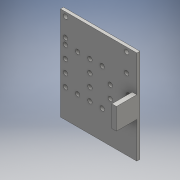
# Autodesk Inventor part: topChassis
Saved by Autodesk Inventor 2016 (Build 200138000, 138)
## iProperties
Created: 2016-05-01
Part Number: topChassis
Material: Generic
Document SubType Name: Modeling
Designer: mkepler
Density: 1 g/cm^3
Appearance: Default
Author: mkepler
Autodesk Inventor part; units mm, degrees
ref_plane "YZ Plane" through (0, 0, 0) normal (1, 0, 0) x (0, 1, 0)
ref_plane "XZ Plane" through (0, 0, 0) normal (0, 1, 0) x (-1, 0, 0)
ref_plane "XY Plane" through (0, 0, 0) normal (0, 0, 1) x (1, 0, 0)
sketch "Sketch1" plane through (0, 0, 0) normal (0, 1, 0) x (-1, 0, 0)
  line L0 (0, 0) -> (75, 0)
  line L1 (75, 0) -> (75, -92)
  line L2 (75, -92) -> (0, -92)
  line L3 (0, -92) -> (0, 0)
  line L4 (75, -46) -> (0, -46)
  circle A0 centre (70, -64) radius 2.175
  circle A1 centre (70, -28) radius 2.175
  circle A2 centre (58, -28) radius 2.175
  circle A3 centre (58, -64) radius 2.175
  circle A4 centre (46, -28) radius 2.175
  circle A5 centre (46, -64) radius 2.175
  circle A6 centre (34, -28) radius 2.175
  circle A7 centre (34, -64) radius 2.175
  dimension "d0" = 75
  dimension "d1" = 92
  dimension "d6" = 4.35
  dimension "d7" = 18
  dimension "d8" = 4.35
  dimension "d9" = 18
  dimension "d10" = 4.35
  dimension "d11" = 12
  dimension "d12" = 4.35
  dimension "d13" = 4.35
  dimension "d14" = 12
  dimension "d15" = 4.35
  dimension "d16" = 4.35
  dimension "d17" = 12
  dimension "d18" = 4.35
  dimension "d19" = 12
  dimension "d20" = 12
  dimension "d21" = 12
  constraints: 10 end point, 8 centre point, 2 midpoint, 2 parallel, 1 horizontal, 1 perpendicular
  measures "d0" distance of L1.end L2.end
  measures "d1" distance of L0.end L1.end
  measures "d6" diameter of A0
  measures "d7" distance from line of L4 A0.centre
  measures "d8" diameter of A1
  measures "d9" distance from line of L4 A1.centre
  measures "d10" diameter of A2
  measures "d11" distance of A2.centre A1.centre
  measures "d12" diameter of A3
  measures "d13" diameter of A4
  measures "d14" distance of A4.centre A2.centre
  measures "d15" diameter of A5
  measures "d16" diameter of A6
  measures "d17" distance of A4.centre A6.centre
  measures "d18" diameter of A7
  measures "d19" distance of A3.centre A0.centre
  measures "d20" distance of A5.centre A3.centre
  measures "d21" distance of A7.centre A5.centre
extrude "Extrusion1" add sketch "Sketch1" along normal blind 3
sketch "Sketch3" plane through (0, 0, 0) normal (0, -1, 0) x (1, 0, 0)
  line L0 (0, 0) -> (0, -92) projected
  line L1 (-4.5, -46) -> (-75, -46)
  line L2 (-75, -92) -> (-75, 0) projected
  line L3 (0, -46) -> (0, -56.5)
  line L4 (0, -56.5) -> (-4.5, -56.5)
  line L5 (-4.5, -56.5) -> (-4.5, -35.5)
  line L6 (-4.5, -35.5) -> (0, -35.5)
  line L7 (0, -56.5) -> (0, -35.5)
  dimension "d24" = 10.5
  dimension "d25" = 4.5
  dimension "d26" = 21
  constraints: 12 end point, 3 midpoint, 2 perpendicular, 2 point on line, 1 collinear, 1 vertical
  measures "d24" distance of L3.start L3.end
  measures "d25" distance of L3.end L4.end
  measures "d26" distance of L4.end L5.end
extrude "Extrusion2" add sketch "Sketch3" along normal blind 20
sketch "Sketch5" plane through (0, 3, 0) normal (0, 1, 0) x (1, 0, 0)
  line L0 (0, 0) -> (0, 92) projected
  line L1 (0, 46) -> (-74.4781, 46)
  circle A0 centre (-8, 52) radius 2.175
  circle A1 centre (-8, 40) radius 2.175
  circle A2 centre (-26, 40) radius 2.175
  circle A3 centre (-26, 52) radius 2.175
  circle A4 centre (-70, 52) radius 2.175
  line L2 (-75, 92) -> (-75, 0) projected
  circle A5 centre (-70, 40) radius 2.175
  circle A6 centre (-46, 52) radius 2.175
  circle A7 centre (-46, 40) radius 2.175
  circle A8 centre (-70, 22) radius 2.175
  circle A9 centre (-70, 4) radius 2.175
  circle A10 centre (-70, 28) radius 2.175 projected
  circle A11 centre (-10, 4) radius 2.175
  circle A12 centre (-10, 22) radius 2.175
  dimension "d29" = 4.35
  dimension "d30" = 6
  dimension "d31" = 8
  dimension "d32" = 4.35
  dimension "d33" = 6
  dimension "d34" = 4.35
  dimension "d35" = 18
  dimension "d36" = 4.35
  dimension "d37" = 4.35
  dimension "d38" = 5
  dimension "d39" = 6
  dimension "d40" = 4.35
  dimension "d41" = 5
  dimension "d42" = 4.35
  dimension "d43" = 24
  dimension "d44" = 4.35
  dimension "d45" = 4.35
  dimension "d46" = 4.35
  dimension "d47" = 18
  dimension "d48" = 6
  dimension "d49" = 6
  dimension "d50" = 6
  dimension "d51" = 6
  dimension "d52" = 6
  dimension "d53" = 12
  dimension "d54" = 4.35
  dimension "d55" = 60
  dimension "d56" = 4.35
  constraints: 12 centre point, 2 end point, 1 horizontal, 1 midpoint
  measures "d29" diameter of A0
  measures "d30" distance from line of L1 A0.centre
  measures "d31" distance from line of L0 A0.centre
  measures "d32" diameter of A1
  measures "d33" distance from line of L1 A1.centre
  measures "d34" diameter of A2
  measures "d35" distance of A1.centre A2.centre
  measures "d36" diameter of A3
  measures "d37" diameter of A4
  measures "d38" distance from line of A4.centre L2
  measures "d39" distance from line of L1 A4.centre
  measures "d40" diameter of A5
  measures "d41" distance from line of L2 A5.centre
  measures "d42" diameter of A6
  measures "d43" distance of A6.centre A4.centre
  measures "d44" diameter of A7
  measures "d45" diameter of A8
  measures "d46" diameter of A9
  measures "d47" distance of A9.centre A8.centre
  measures "d48" distance of A10.centre A8.centre
  measures "d49" distance from line of L1 A5.centre
  measures "d50" distance from line of L1 A7.centre
  measures "d51" distance from line of L1 A6.centre
  measures "d52" distance from line of L1 A2.centre
  measures "d53" distance of A2.centre A3.centre
  measures "d54" diameter of A11
  measures "d55" distance of A11.centre A9.centre
  measures "d56" diameter of A12
hole "Hole1" at (-70, 3, -4) at (-70, 3, -22) at (-70, 3, -40) at (-70, 3, -52) at (-46, 3, -52) at (-46, 3, -40) at (-26, 3, -40) at (-10, 3, -22) at (-10, 3, -4) at (-8, 3, -40) at (-26, 3, -52) at (-8, 3, -52) direction (0, -1, 0) diameter 4.35 end through all
body "Solid1"
